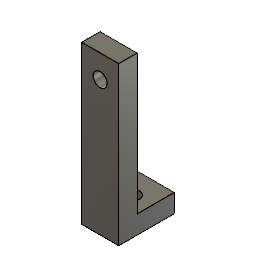
X Axix Belt (Autodesk Fusion 360 design; units mm, degrees)
Autodesk Fusion 360 part; units mm, degrees
sketch "Skizze1" plane through (0, 0, 0) normal (0, 1, 0) x (1, 0, 0)
  line L0 (0, 0) -> (8, 0)
  line L1 (0, 0) -> (0, -12)
  line L2 (8, 0) -> (8, -12)
  line L3 (0, -12) -> (8, -12)
  dimension "d1" = 8
  dimension "d2" = 12
  dimension "d3" = 12
  constraint coincident L0.start L1.start
  constraint horizontal L0
  constraint perpendicular L0 L1
  constraint perpendicular L0 L2
  measures "d1" distance of L0.start L0.end
  measures "d2" distance of L0.start L1.end
  measures "d3" distance of L0.end L2.end
extrude "Extrusion1" add sketch "Skizze1" along normal blind 4
sketch "Skizze2" plane through (0, 4, 0) normal (0, 1, 0) x (-1, 0, 0)
  line L0 (0, 0) -> (0, 12)
  line L1 (0, 12) -> (-8, 12)
  line L2 (-8, 12) -> (-8, 0)
  line L3 (-8, 0) -> (0, 0)
  circle A0 centre (-4, 5) radius 1.5
  dimension "d6" = 3
  measures "d6" diameter of A0
extrude "Extrusion2" cut sketch "Skizze2" against normal blind 15 contours A0
sketch "Skizze3" plane through (0, 4, 0) normal (0, 1, 0) x (-1, 0, 0)
  circle A0 centre (-4, 5) radius 1.5
  line L0 (0, 0) -> (0, 12)
  line L1 (0, 12) -> (-8, 12)
  line L2 (-8, 12) -> (-8, 0)
  line L3 (-8, 0) -> (0, 0)
  line L4 (0, 12) -> (0, 9)
  line L5 (0, 9) -> (0, 8)
  line L6 (0, 8) -> (-8, 8)
  line L7 (-8, 8) -> (-8, 12)
  line L8 (-8, 12) -> (0, 12)
  constraint coincident L0.end L1.start
  constraint coincident L0 L4.end
  constraint perpendicular L1 L4
  constraint coincident L0 L5.end
  constraint parallel L0 L5
  constraint coincident L2 L6.end
  constraint perpendicular L2 L6
  constraint coincident L1.end L2.start
extrude "Extrusion3" add sketch "Skizze3" along normal blind 30 contours L0 L1 L2 L4 L5 L6 L7 L8
sketch "Skizze4" plane through (0, 0, 12) normal (0, 0, 1) x (1, 0, 0)
  line L0 (0, 0) -> (8, 0)
  line L1 (8, 0) -> (8, 34)
  line L2 (8, 34) -> (0, 34)
  line L3 (0, 34) -> (0, 0)
  line L4 (0, 34) -> (0, 29)
  line L5 (0, 29) -> (4, 29)
  circle A0 centre (4, 29) radius 1.5
  dimension "d11" = 3
  constraint coincident L2.end L3.start
  constraint coincident L3 L4.end
  constraint perpendicular L2 L4
  constraint perpendicular L3 L5
  constraint coincident L5.end A0.centre
  measures "d11" diameter of A0
extrude "Extrusion4" cut sketch "Skizze4" against normal blind 21 contours A0
